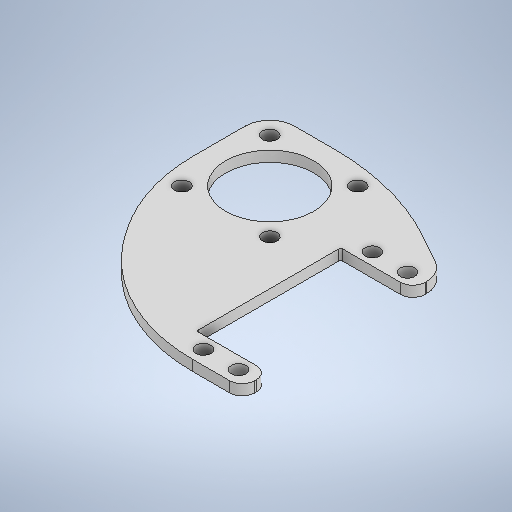
# Autodesk Inventor part: plyka zawor servo
Saved by Autodesk Inventor 2025 (Build 290162000, 162)
## iProperties
Created: 2025-04-09
Part Number: plyka zawor servo
Material: Ogólny
Document SubType Name: Modeling
Designer: Dell
Density: 1 g/cm^3
Appearance: Domyślna
Author: Dell
Autodesk Inventor part; units mm, degrees
ref_plane "YZ Plane" through (0, 0, 0) normal (1, 0, 0) x (0, 1, 0)
ref_plane "XZ Plane" through (0, 0, 0) normal (0, 1, 0) x (-1, 0, 0)
ref_plane "XY Plane" through (0, 0, 0) normal (0, 0, 1) x (1, 0, 0)
sketch "Szkic1" plane through (0, 0, 0) normal (0, 1, 0) x (-1, 0, 0)
  circle A0 centre (0, 0) radius 12.5
  line L0 (-12.5, 12.5) -> (12.5, 12.5)
  line L1 (12.5, 12.5) -> (12.5, -12.5)
  line L2 (12.5, -12.5) -> (-12.5, -12.5)
  line L3 (-12.5, -12.5) -> (-12.5, 12.5)
  line L4 (-12.5, 12.5) -> (12.5, -12.5) construction
  line L5 (12.5, 12.5) -> (-12.5, -12.5) construction
  circle A1 centre (12.5, -12.5) radius 2.1
  circle A2 centre (-12.5, -12.5) radius 2.1
  circle A3 centre (-12.5, 12.5) radius 2.1
  circle A4 centre (12.5, 12.5) radius 2.1
  circle A5 centre (0, 0) radius 50.5
  line L6 (-25, 3.4426) -> (25, 3.4426)
  line L7 (25, 3.4426) -> (25, -3.4426)
  line L8 (25, -3.4426) -> (-25, -3.4426)
  line L9 (-25, -3.4426) -> (-25, 3.4426)
  line L10 (-25, 3.4426) -> (25, -3.4426) construction
  line L11 (25, 3.4426) -> (-25, -3.4426) construction
  circle A6 centre (-35.7881, 35.6295) radius 3
  line L12 (-35.7881, 38.6295) -> (-35.7881, 45.6295)
  line L13 (-35.7881, 32.6295) -> (-35.7881, 5.6295)
  line L14 (-35.7881, 5.6295) -> (-35.7881, 25.6295)
  line L15 (-45.7881, 45.6295) -> (-25.7881, 45.6295)
  line L16 (-25.7881, 45.6295) -> (-25.7881, 5.6295)
  line L17 (-25.7881, 5.6295) -> (-45.7881, 5.6295)
  line L18 (-45.7881, 5.6295) -> (-45.7881, 45.6295)
  line L19 (-45.7881, 45.6295) -> (-25.7881, 5.6295) construction
  line L20 (-25.7881, 45.6295) -> (-45.7881, 5.6295) construction
  line L21 (-40.7881, 49.6295) -> (-30.7881, 49.6295)
  line L22 (-30.7881, 49.6295) -> (-30.7881, 1.6295)
  line L23 (-30.7881, 1.6295) -> (-40.7881, 1.6295)
  line L24 (-40.7881, 1.6295) -> (-40.7881, 49.6295)
  line L25 (-40.7881, 49.6295) -> (-30.7881, 1.6295) construction
  line L26 (-30.7881, 49.6295) -> (-40.7881, 1.6295) construction
  circle A7 centre (-30.7881, 1.6295) radius 2.1
  circle A8 centre (-40.7881, 1.6295) radius 2.1
  circle A9 centre (-40.7881, 49.6295) radius 2.1
  circle A10 centre (-30.7881, 49.6295) radius 2.1
  line L27 (-46.2881, 46.1295) -> (-25.2881, 46.1295)
  line L28 (-25.2881, 46.1295) -> (-25.2881, 5.1295)
  line L29 (-25.2881, 5.1295) -> (-46.2881, 5.1295)
  line L30 (-46.2881, 5.1295) -> (-46.2881, 46.1295)
  line L31 (-46.2881, 46.1295) -> (-25.2881, 5.1295) construction
  line L32 (-25.2881, 46.1295) -> (-46.2881, 5.1295) construction
  line L33 (-35.7881, 45.6295) -> (-35.7881, 53.6295)
  line L34 (-35.7881, 53.6295) -> (-45.7881, 53.6295)
  line L35 (-45.7881, 53.6295) -> (-45.7881, 46.1295)
  line L36 (-35.7881, 53.6295) -> (-5.7881, 53.6295)
  line L37 (-18.25, 18.25) -> (18.25, 18.25)
  line L38 (18.25, 18.25) -> (18.25, -18.25)
  line L39 (18.25, -18.25) -> (-18.25, -18.25)
  line L40 (-18.25, -18.25) -> (-18.25, 18.25)
  line L41 (-18.25, 18.25) -> (18.25, -18.25) construction
  line L42 (18.25, 18.25) -> (-18.25, -18.25) construction
  line L43 (18.25, 18.25) -> (-5.7881, 53.6295)
  line L44 (-45.7881, 5.1295) -> (-45.7881, -2.8705)
  line L45 (-45.7881, -2.8705) -> (-18.25, -18.25)
  dimension "d9" = 101
  dimension "d0" = 25
  dimension "d1" = 25
  dimension "d2" = 25
  dimension "d3" = 4.2
  dimension "d4" = 4.2
  dimension "d5" = 4.2
  dimension "d6" = 4.2
  dimension "d13" = 50
  dimension "d17" = 6
  dimension "d18" = 7
  dimension "d19" = 27
  dimension "d20" = 20
  dimension "d21" = 20
  dimension "d22" = 40
  dimension "d23" = 10
  dimension "d24" = 48
  dimension "d25" = 4.2
  dimension "d26" = 4.2
  dimension "d27" = 4.2
  dimension "d28" = 4.2
  dimension "d29" = 21
  dimension "d30" = 41
  dimension "d31" = 8
  dimension "d32" = 10
  dimension "d33" = 30
  dimension "d34" = 36.5
  dimension "d35" = 36.5
  dimension "d36" = 8
  constraints: 92 end point, 13 parallel, 12 midpoint, 10 centre point, 10 coincident, 7 horizontal, 7 perpendicular, 4 point on line, 3 vertical, 2 point on circle, 3 other
  measures "d0" diameter of A0
  measures "d1" distance of L1.end L2.end
  measures "d2" distance of L0.end L1.end
  measures "d3" diameter of A1
  measures "d4" diameter of A2
  measures "d5" diameter of A3
  measures "d6" diameter of A4
  measures "d13" distance of L7.end L8.end
  measures "d17" diameter of A6
  measures "d18" distance of L12.start L12.end
  measures "d19" distance of L13.start L13.end
  measures "d20" distance of L13.end L14.end
  measures "d21" distance of L16.end L17.end
  measures "d22" distance of L15.end L16.end
  measures "d23" distance of L22.end L23.end
  measures "d24" distance of L21.end L22.end
  measures "d25" diameter of A7
  measures "d26" diameter of A8
  measures "d27" diameter of A9
  measures "d28" diameter of A10
  measures "d29" distance of L28.end L29.end
  measures "d30" distance of L27.end L28.end
  measures "d31" distance of L12.end L33.end
  measures "d32" distance of L33.end L34.end
  measures "d33" distance of L33.end L36.end
  measures "d34" distance of L38.end L39.end
  measures "d35" distance of L37.end L38.end
  measures "d36" distance of L44.start L44.end
extrude "Wyciągnięcie proste1" add sketch "Szkic1" along normal blind 3 contours L1 L8 A0 | A0 L6 L1 | L1 L6 L38 L8 | A0 L0 A4 L1 L6 | L8 L1 A1 L2 A0 | L1 A4 L0 A3 L3 L6 L40 L37 L38 | L8 L38 L39 L40 L3 A2 L2 A1 L1 | A0 L6 L3 A3 L0 | A0 L3 L6 | L2 A2 L3 L8 A0 | L8 L3 A0 | L3 L8 L40 L6 | L37 L40 L6 L9 L8 L45 L44 L29 L24 A8 L23 A7 L22 L28 A5 L43 | L40 L8 L9 L6 | A5 L28 L27 L22 A10 L21 L33 L36 L43 | L33 L21 A9 L24 L27 L35 L34 | L27 L33 L21 A10 L22 | L22 A7 L23 A8 L24 L29 | L33 L27 L24 A9 L21
fillet "Zaokrąglenie1" radius 0.5 2 edges at (25.2881, 1.5, 5.1295) (25.2881, 1.5, 46.1295)
fillet "Zaokrąglenie3" radius 3.5 3 edges at (45.7881, 1.5, 5.1295) (45.7881, 1.5, 46.1295) (45.7881, 1.5, 53.6295)
fillet "Zaokrąglenie4" radius 7 1 edges at (45.7881, 1.5, -2.8705)
fillet "Zaokrąglenie5" radius 70 1 edges at (18.25, 1.5, -18.25)
fillet "Zaokrąglenie6" radius 49 1 edges at (5.7881, 1.5, 53.6295)
fillet "Zaokrąglenie7" radius 49 1 edges at (-18.25, 1.5, 18.25)
fillet "Zaokrąglenie8" radius 7 1 edges at (-18.25, 1.5, -18.25)
